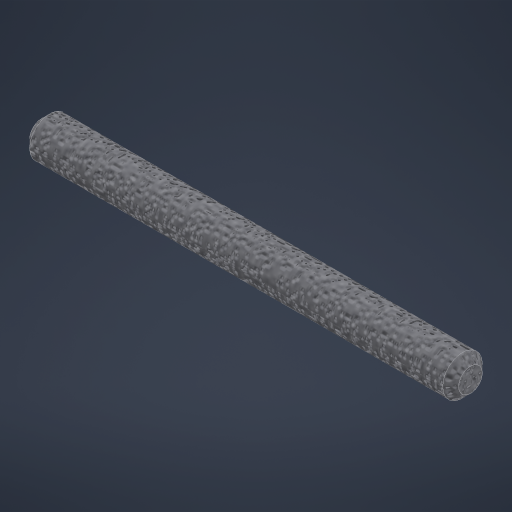
# Autodesk Inventor part: Barrel Resting Pin
Saved by Autodesk Inventor 2024.1 (Build 281209000, 209)
## iProperties
Created: 2023-10-23
Part Number: Barrel Resting Pin
Material: Iron, Cast
Document SubType Name: Modeling
Designer: LEGION SMIT
Density: 7.15 g/cm^3
Appearance: Iron - Cast
Author: LEGION SMIT
Autodesk Inventor part; units mm, degrees
ref_plane "YZ Plane" through (0, 0, 0) normal (1, 0, 0) x (0, 1, 0)
ref_plane "XZ Plane" through (0, 0, 0) normal (0, 1, 0) x (-1, 0, 0)
ref_plane "XY Plane" through (0, 0, 0) normal (0, 0, 1) x (1, 0, 0)
sketch "Sketch1" plane through (0, 0, 0) normal (1, 0, 0) x (0, 1, 0)
  circle A0 centre (0, 0) radius 2.5
  dimension "d0" = 5
  constraints: 1 centre point, 1 coincident
  measures "d0" diameter of A0
extrude "Extrusion1" add sketch "Sketch1" against normal blind 54
chamfer "Chamfer1" distance 1 angle 45 2 edges at (-54, -2.5, 0) (0, -2.5, 0)
body "Solid1"
